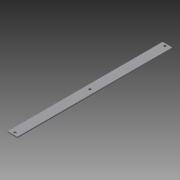
# Autodesk Inventor part: Jack FlatStock
Saved by Autodesk Inventor 2015 (Build 190159000, 159)
## iProperties
Created: 2017-01-05
Part Number: Jack FlatStock
Material: Generic
Document SubType Name: Modeling
Designer: ps2du
Density: 1 g/cm^3
Appearance: Default
Author: ps2du
Autodesk Inventor part; units mm, degrees
ref_plane "YZ Plane" through (0, 0, 0) normal (1, 0, 0) x (0, 1, 0)
ref_plane "XZ Plane" through (0, 0, 0) normal (0, 1, 0) x (-1, 0, 0)
ref_plane "XY Plane" through (0, 0, 0) normal (0, 0, 1) x (1, 0, 0)
sketch "Sketch1" plane through (0, 0, 0) normal (0, 0, 1) x (1, 0, 0)
  line L0 (0, 0) -> (25.4, 0)
  line L1 (25.4, 0) -> (25.4, 3.175)
  line L2 (25.4, 3.175) -> (0, 3.175)
  line L3 (0, 3.175) -> (0, 0)
  dimension "d0" = 25.4
  dimension "d1" = 3.175
  constraints: 8 end point, 2 parallel, 1 horizontal, 1 perpendicular
  measures "d0" distance of L2.end L1.end
  measures "d1" distance of L1.end L0.end
extrude "Extrusion1" add sketch "Sketch1" along normal blind 406.4
sketch "Sketch2" plane through (0, 3.175, 0) normal (0, 1, 0) x (1, 0, 0)
  line L0 (0, 0) -> (25.4, 0)
  line L1 (0, 0) -> (25.4, 0) projected
  line L2 (12.7, 0) -> (12.7, -406.4)
  line L3 (0, -406.4) -> (25.4, -406.4)
  line L4 (12.7, 0) -> (12.7, -6.35)
  line L5 (12.7, -406.4) -> (12.7, -400.05)
  line L6 (12.7, -406.4) -> (12.7, -203.2)
  dimension "d4" = 6.35
  dimension "d5" = 6.35
  dimension "d6" = 203.2
  constraints: 12 end point, 3 coincident, 3 midpoint, 2 point on line, 1 collinear, 1 horizontal, 1 vertical
  measures "d4" distance of L2.start L4.end
  measures "d5" distance of L2.end L5.end
  measures "d6" distance of L2.end L6.end
hole "Hole1" at (12.7, 3.175, 6.35) at (12.7, 3.175, 400.05) at (12.7, 3.175, 203.2) direction (0, -1, 0) diameter 6.35 end through all
body "Solid1"
